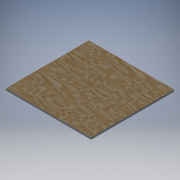
# Autodesk Inventor part: Plywood Base - TBone
Saved by Autodesk Inventor 2018.2 (Build 222227000, 227)
## iProperties
Created: 2018-02-01
Part Number: Plywood Base - TBone
Material: Generic
Document SubType Name: Modeling
Designer: owner
Density: 1 g/cm^3
Appearance: Default
Author: owner
Autodesk Inventor part; units mm, degrees
ref_plane "YZ Plane" through (0, 0, 0) normal (1, 0, 0) x (0, 1, 0)
ref_plane "XZ Plane" through (0, 0, 0) normal (0, 1, 0) x (-1, 0, 0)
ref_plane "XY Plane" through (0, 0, 0) normal (0, 0, 1) x (1, 0, 0)
sketch "Sketch1" plane through (0, 0, 0) normal (0, 0, 1) x (1, 0, 0)
  line L0 (0, 0) -> (762, 0)
  line L1 (762, 0) -> (762, 19.05)
  line L2 (762, 19.05) -> (0, 19.05)
  line L3 (0, 19.05) -> (-43.4138, 19.05)
  line L4 (-43.4138, 0) -> (0, 0)
  line L5 (-43.815, 19.05) -> (-43.815, 23.2664)
  line L6 (-43.4138, 19.05) -> (-43.815, 19.05)
  line L7 (-43.815, 19.05) -> (-43.815, 0)
  line L8 (-43.815, 0) -> (-43.4138, 0)
  dimension "d0" = 762
  dimension "d1" = 19.05
  constraints: 18 end point, 2 horizontal, 2 parallel, 2 perpendicular, 2 vertical, 3 other
  measures "d0" distance of L0.start L0.end
  measures "d1" distance of L0.end L1.end
extrude "Extrusion1" add sketch "Sketch1" against normal blind 784.8092
body "Solid1"
